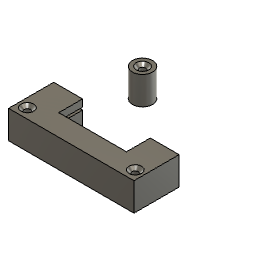
drzak_ridici_desky_v1 (Autodesk Fusion 360 design; units mm, degrees)
Autodesk Fusion 360 part; units mm, degrees
sketch "Sketch1" plane through (0, 0, 0) normal (0, 1, 0) x (1, 0, 0)
  line L0 (0, 0) -> (70, 0)
  line L1 (70, 0) -> (70, 50)
  line L2 (70, 50) -> (0, 50)
  line L3 (0, 50) -> (0, 0)
  dimension "d1" = 70
  dimension "d2" = 50
  constraint horizontal L0
  constraint vertical L1
  constraint horizontal L2
  constraint vertical L3
  constraint coincident L0.start L3.end
  measures "d1" distance of L0.start L0.end
  measures "d2" distance of L0.start L2.end
extrude "Extrude1" add sketch "Sketch1" along normal blind 1.4 makes body 1
sketch "Sketch2" plane through (0, 0, 0) normal (0, 1, 0) x (1, 0, 0)
  line L0 (0, 0) -> (70, 0)
  line L1 (70, 0) -> (70, 2)
  line L2 (70, 2) -> (0, 2)
  line L3 (0, 2) -> (0, 0)
  line L4 (0, 0) -> (8, 0)
  line L5 (8, 0) -> (8, 21)
  line L6 (8, 21) -> (0, 21)
  line L7 (0, 21) -> (0, 0)
  line L8 (70, 0) -> (62, 0)
  line L9 (62, 0) -> (62, 21)
  line L10 (62, 21) -> (70, 21)
  line L11 (70, 21) -> (70, 0)
  line L12 (0, 0) -> (-15, 0)
  line L13 (-15, 0) -> (-15, -15)
  line L14 (-15, -15) -> (0, -15)
  line L15 (0, -15) -> (0, 0)
  line L16 (-15, -15) -> (85, -15)
  line L17 (85, -15) -> (85, 21)
  line L18 (85, 21) -> (-15, 21)
  line L19 (-15, 21) -> (-15, -15)
  dimension "d5" = 70
  dimension "d6" = 2
  dimension "d7" = 8
  dimension "d8" = 21
  dimension "d9" = 8
  dimension "d10" = 21
  dimension "d11" = 15
  dimension "d12" = 15
  dimension "d13" = 100
  dimension "d14" = 36
  constraint horizontal L0
  constraint vertical L1
  constraint horizontal L2
  constraint vertical L3
  constraint coincident L0.start L3.end
  constraint horizontal L4
  constraint vertical L5
  constraint horizontal L6
  constraint vertical L7
  constraint horizontal L8
  constraint vertical L9
  constraint horizontal L10
  constraint vertical L11
  constraint horizontal L12
  constraint vertical L13
  constraint horizontal L14
  constraint vertical L15
  constraint horizontal L16
  constraint vertical L17
  constraint horizontal L18
  constraint vertical L19
  measures "d5" distance of L0.start L0.end
  measures "d6" distance of L0.start L2.end
  measures "d7" distance of L0.start L4.end
  measures "d8" distance of L0.start L6.end
  measures "d9" distance of L0.end L8.end
  measures "d10" distance of L0.end L10.end
  measures "d11" distance of L0.start L12.end
  measures "d12" distance of L0.start L14.end
  measures "d13" distance of L13.end L16.end
  measures "d14" distance of L13.end L18.end
extrude "Extrude2" add sketch "Sketch2" along normal up to surface (1.4 mm away) separate body contours L0 L2 L3 L4 L5 L7 | L3 L7 L12 L18 L19 | L12 L13 L14 L15 L16 L19 | L0 L1 L4 L8 L11 L15 L16 L17 L18 | L0 L2 L5 L9 | L2 L5 L6 L7 L18 | L0 L1 L2 L8 L9 L11 | L2 L9 L10 L11 L18 makes body 2
extrude "Extrude3" add 1 faces at (77.3333, 1.4, -2.6667) along direction (0, 1, 0) blind 6 on bodies 2 bodies 2
extrude "Extrude4" add 1 faces at (-7.3333, 0, -2.6667) along direction (0, -1, 0) blind 15 on bodies 2 bodies 2
combine "Combine1" operation cut target body 2 tool bodies 1 keep tools
extrude "Extrude5" cut 1 faces at (2.6667, 1.4, -7.6667) along direction (0, 1, 0) blind 0.3 on bodies 2 bodies 2
extrude "Extrude6" cut 1 faces at (2.6667, 0, -7.6667) along direction (0, -1, 0) blind 0.3 on bodies 2 bodies 2
extrude "Extrude7" cut 1 faces at (0, 0.3667, -7) along direction (-1, 0, 0) blind 0.4 on bodies 2 bodies 2
extrude "Extrude8" cut 1 faces at (70, 1.0333, -7) along direction (1, 0, 0) blind 0.4 on bodies 2 bodies 2
sketch "Sketch3" plane through (0, 7.4, 0) normal (0, 1, 0) x (-1, 0, 0)
  line L0 (-62, -21) -> (-62, -2)
  line L1 (-62, -2) -> (-8, -2)
  line L2 (-8, -2) -> (-8, -21)
  line L3 (-8, -21) -> (15, -21)
  line L4 (15, -21) -> (15, 15)
  line L5 (15, 15) -> (-85, 15)
  line L6 (-85, 15) -> (-85, -21)
  line L7 (-85, -21) -> (-62, -21)
  line L8 (15, -21) -> (8, -21)
  line L9 (8, -21) -> (8, 7)
  line L10 (8, 7) -> (15, 7)
  line L11 (15, 7) -> (15, -21)
  line L12 (-85, -21) -> (-78, -21)
  line L13 (-78, -21) -> (-78, 7)
  line L14 (-78, 7) -> (-85, 7)
  line L15 (-85, 7) -> (-85, -21)
  dimension "d29" = 7
  dimension "d30" = 28
  dimension "d31" = 7
  dimension "d32" = 28
  constraint horizontal L8
  constraint vertical L9
  constraint horizontal L10
  constraint vertical L11
  constraint coincident L3.end L4.start
  constraint horizontal L12
  constraint vertical L13
  constraint horizontal L14
  constraint vertical L15
  constraint coincident L6.end L7.start
  measures "d29" distance of L3.end L8.end
  measures "d30" distance of L3.end L10.end
  measures "d31" distance of L6.end L12.end
  measures "d32" distance of L6.end L14.end
hole "Hole1" at (-8, 7.4, 7) at (78, 7.4, 7) direction (0, -1, 0) diameter 5 depth 40 tip angle 118 countersink diameter 10 countersink angle 90 bodies 2
sketch "Sketch4" plane through (0, 0, 0) normal (0, 1, 0) x (1, 0, 0)
  circle A0 centre (9.3748, 67.4518) radius 8
  dimension "d38" = 16
  measures "d38" diameter of A0
extrude "Extrude9" add sketch "Sketch4" against normal up to surface (15 mm away) separate body makes body 3
extrude "Extrude10" add 1 faces at (7.0259, 0, -69.325) along direction (0, 1, 0) up to surface (7.4 mm away) on bodies 3 bodies 3
hole "Hole2" at (9.3748, 7.4, -67.4518) direction (0, -1, 0) diameter 5 depth 40 tip angle 118 countersink diameter 10 countersink angle 90 bodies 3
hidden bodies 1
equation "d13 = 85.000 mm + 15 mm"
